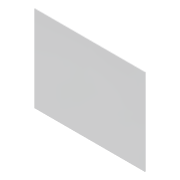
# Autodesk Inventor part: cellSTORM_laserbeam_meander_chip
Saved by Autodesk Inventor 2019.4 (Build 234330000, 330)
## iProperties
Created: 2020-09-02
Part Number: cellSTORM_laserbeam_meander_chip
Material: Generic
Document SubType Name: Modeling
Designer: diederichbenedict
Density: 1 g/cm^3
Appearance: Polycarbonate - Clear
Author: diederichbenedict
Autodesk Inventor part; units mm, degrees
ref_plane "YZ Plane" through (0, 0, 0) normal (1, 0, 0) x (0, 1, 0)
ref_plane "XZ Plane" through (0, 0, 0) normal (0, 1, 0) x (-1, 0, 0)
ref_plane "XY Plane" through (0, 0, 0) normal (0, 0, 1) x (1, 0, 0)
sketch "Sketch1" plane through (0, 0, 0) normal (0, 0, 1) x (1, 0, 0)
  line L0 (-1.5, -25) -> (-0.2518, -25) projected
  line L1 (26.9054, -25) -> (-90.2508, -25)
  line L2 (-90.2508, -25) -> (-90.2508, 84.6714)
  line L3 (-90.2508, 84.6714) -> (26.9054, 84.6714)
  line L4 (26.9054, 84.6714) -> (26.9054, -25)
  point P0 (0, 0)
  constraints: 8 end point, 2 parallel, 1 horizontal, 1 perpendicular
extrude "Extrusion1" add sketch "Sketch1" along normal blind 1
sketch "Sketch2" plane through (0, 0, 0) normal (0, 0, -1) x (-1, 0, 0)
  point P0 (0, 0)
sketch "Sketch3" plane through (0, 0, 0) normal (0, 0, -1) x (-1, 0, 0)
  line L0 (-26.9054, -25) -> (90.2508, -25) projected
  line L1 (90.2508, -25) -> (90.2508, 84.6714) projected
  line L2 (90.2508, 84.6714) -> (-26.9054, 84.6714) projected
  line L3 (-26.9054, 84.6714) -> (-26.9054, -25) projected
  line L4 (-26.9054, -25) -> (-26.9054, 84.6714) projected
  line L5 (90.2508, -25) -> (-26.9054, -25) projected
  line L6 (-26.9054, 84.6714) -> (-21.9054, 84.6714)
  line L7 (-21.9054, 84.6714) -> (-21.9054, -25)
  line L8 (-21.9054, -25) -> (-26.9054, -25)
  line L9 (-26.9054, -25) -> (-26.9054, 84.6714)
  line L10 (-12.9054, 84.6714) -> (-7.9054, 84.6714)
  line L11 (-7.9054, 84.6714) -> (-7.9054, -25)
  line L12 (-7.9054, -25) -> (-12.9054, -25)
  line L13 (-12.9054, -25) -> (-12.9054, 84.6714)
  line L14 (1.0946, 84.6714) -> (6.0946, 84.6714)
  line L15 (6.0946, 84.6714) -> (6.0946, -25)
  line L16 (6.0946, -25) -> (1.0946, -25)
  line L17 (1.0946, -25) -> (1.0946, 84.6714)
  line L18 (15.0946, 84.6714) -> (20.0946, 84.6714)
  line L19 (20.0946, 84.6714) -> (20.0946, -25)
  line L20 (20.0946, -25) -> (15.0946, -25)
  line L21 (15.0946, -25) -> (15.0946, 84.6714)
  line L22 (29.0946, 84.6714) -> (34.0946, 84.6714)
  line L23 (34.0946, 84.6714) -> (34.0946, -25)
  line L24 (34.0946, -25) -> (29.0946, -25)
  line L25 (29.0946, -25) -> (29.0946, 84.6714)
  line L26 (43.0946, 84.6714) -> (48.0946, 84.6714)
  line L27 (48.0946, 84.6714) -> (48.0946, -25)
  line L28 (48.0946, -25) -> (43.0946, -25)
  line L29 (43.0946, -25) -> (43.0946, 84.6714)
  line L30 (57.0946, 84.6714) -> (62.0946, 84.6714)
  line L31 (62.0946, 84.6714) -> (62.0946, -25)
  line L32 (62.0946, -25) -> (57.0946, -25)
  line L33 (57.0946, -25) -> (57.0946, 84.6714)
  line L34 (71.0946, 84.6714) -> (76.0946, 84.6714)
  line L35 (76.0946, 84.6714) -> (76.0946, -25)
  line L36 (76.0946, -25) -> (71.0946, -25)
  line L37 (71.0946, -25) -> (71.0946, 84.6714)
  line L38 (85.0946, 84.6714) -> (90.0946, 84.6714)
  line L39 (90.0946, 84.6714) -> (90.0946, -25)
  line L40 (90.0946, -25) -> (85.0946, -25)
  line L41 (85.0946, -25) -> (85.0946, 84.6714)
  point P0 (0, 0)
  point P1 (-12.9054, -25)
  point P2 (1.0946, -25)
  point P3 (15.0946, -25)
  point P4 (29.0946, -25)
  point P5 (43.0946, -25)
  point P6 (57.0946, -25)
  point P7 (71.0946, -25)
  dimension "d2" = 5
  dimension "d5" = 14
  constraints: 72 end point, 2 horizontal, 2 parallel, 1 perpendicular, 1 point on line, 72 other
  measures "d2" distance of L7.end L8.end
  measures "d5" distance of L0.start point (-12.905, -25)
extrude "Extrusion2" add sketch "Sketch3" along normal blind 1 contours L3 L2 L7 L0 | L13 L2 L11 L0 | L17 L2 L15 L0 | L21 L2 L19 L0 | L25 L2 L23 L0 | L29 L2 L27 L0 | L33 L2 L31 L0 | L37 L2 L35 L0 | L41 L2 L39 L0
sketch "Sketch4" plane through (0, 0, -1) normal (0, 0, -1) x (-1, 0, 0)
  line L0 (-1.5, 25) -> (58.5, 25) projected
  line L1 (-1.5, -25) -> (-1.5, 25) projected
  line L2 (-0.2518, -25) -> (-1.5, -25) projected
  line L3 (0.2518, -25) -> (-0.2518, -25) projected
  line L4 (1.5, -25) -> (0.2518, -25) projected
  line L5 (1.5, 22) -> (1.5, -25) projected
  line L6 (1.5, 22) -> (61.5, 22) projected
  line L7 (61.5, 22) -> (61.5, 35) projected
  line L8 (61.5, 35) -> (1.5, 35) projected
  line L9 (1.5, 35) -> (1.5, 42) projected
  line L10 (1.5, 42) -> (61.5, 42) projected
  line L11 (61.5, 42) -> (61.5, 55) projected
  line L12 (61.5, 55) -> (1.5, 55) projected
  line L13 (1.5, 55) -> (1.5, 62) projected
  line L14 (1.5, 62) -> (61.5, 62) projected
  line L15 (61.5, 62) -> (61.5, 75) projected
  line L16 (61.5, 75) -> (1.5, 75) projected
  line L17 (1.5, 75) -> (1.5, 85) projected
  line L18 (1.5, 85) -> (-1.5, 85) projected
  line L19 (-1.5, 85) -> (-1.5, 72) projected
  line L20 (-1.5, 72) -> (58.5, 72) projected
  line L21 (58.5, 72) -> (58.5, 65) projected
  line L22 (58.5, 65) -> (-1.5, 65) projected
  line L23 (-1.5, 65) -> (-1.5, 52) projected
  line L24 (-1.5, 52) -> (58.5, 52) projected
  line L25 (58.5, 52) -> (58.5, 45) projected
  line L26 (58.5, 45) -> (-1.5, 45) projected
  line L27 (-1.5, 45) -> (-1.5, 32) projected
  line L28 (-1.5, 32) -> (58.5, 32) projected
  line L29 (58.5, 32) -> (58.5, 25) projected
  point P0 (0, 0)
extrude "Extrusion3" cut sketch "Sketch4" against normal up to surface (1 mm away)
body "Solid1"
